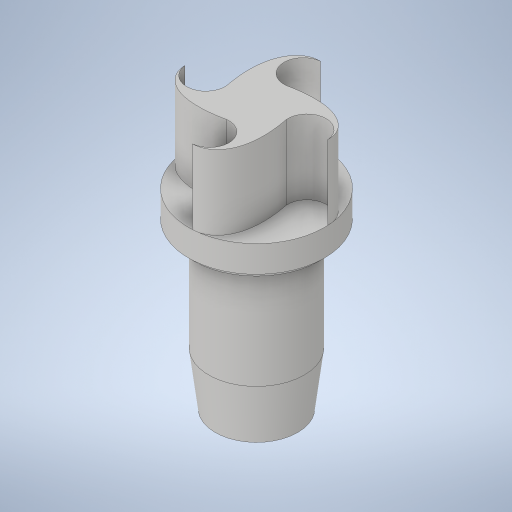
# Autodesk Inventor part: 1.3mm_uncorrected
Saved by Autodesk Inventor 2023.1 (Build 271208000, 208)
## iProperties
Created: 2020-02-22
Part Number: 1.3mm_uncorrected
Material: Générique
Document SubType Name: Modeling
Designer: kongooi
Density: 1 g/cm^3
Appearance: Par défaut
Author: kongooi
Autodesk Inventor part; units mm, degrees
ref_plane "YZ Plane" through (0, 0, 0) normal (1, 0, 0) x (0, 1, 0)
ref_plane "XZ Plane" through (0, 0, 0) normal (0, 1, 0) x (-1, 0, 0)
ref_plane "XY Plane" through (0, 0, 0) normal (0, 0, 1) x (1, 0, 0)
sketch "Sketch2" plane through (0, 0, 0) normal (0, 1, 0) x (-1, 0, 0)
  line L0 (-0.279026, 0.279026) -> (0.279026, -0.279026) construction
  line L1 (0.279026, 0.279026) -> (-0.279026, -0.279026) construction
  spline S0 degree 4 poles (-0.639115, -0.03369) (-0.634493, -0.132924) (-0.626677, -0.000796) (-0.683231, -0.424589) (0.000022, -0.278707) knots 0 0 0 0 0 1 1 1 1 1
  spline S1 degree 4 poles (0.036579, -0.638954) (0.128591, -0.633029) (0.015735, -0.629627) (0.410949, -0.676473) (0.279026, 0) knots 0 0 0 0 0 1 1 1 1 1
  spline S2 degree 4 poles (-0.036525, 0.638959) (-0.129118, 0.634798) (-0.010002, 0.617131) (-0.415936, 0.686883) (-0.279026, 0) knots 0 0 0 0 0 1 1 1 1 1
  spline S3 degree 4 poles (0.638959, 0.036525) (0.634795, 0.128622) (0.619543, 0.004623) (0.682049, 0.421677) (0, 0.279026) knots 0 0 0 0 0 1 1 1 1 1
  arc A0 (-0.639115, -0.03369) -> (-0.279026, 0) centre (-0.45907, -0.016845) ccw
  arc A1 (0.036579, -0.638954) -> (0.000022, -0.278707) centre (0.0183, -0.45883) ccw
  arc A2 (0.638959, 0.036525) -> (0.279026, 0) centre (0.458993, 0.018263) ccw
  arc A3 (-0.036525, 0.638959) -> (0, 0.279026) centre (-0.018263, 0.458993) ccw
  circle A4 centre (0, 0) radius 0.64
  point P0 (0.072027, -0.636054)
  point P1 (0.088403, -0.633939)
  point P2 (0.119628, -0.625229)
  point P3 (-0.071713, 0.635654)
  point P4 (-0.087466, 0.632637)
  point P5 (-0.11823, 0.62326)
  point P6 (0.635846, 0.070961)
  point P7 (0.633021, 0.08595)
  point P8 (0.62382, 0.11598)
  point P9 (-0.636387, -0.071601)
  point P10 (-0.634237, -0.087213)
  point P11 (-0.625654, -0.117837)
  dimension "d14" = 1.28
  constraints: 8 point on circle, 4 centre point, 4 end point, 2 midpoint, 1 coincident, 31 other
sketch "Sketch2 outline for Extrusion1" plane through (0, 0, 0) normal (0, 1, 0) x (-1, 0, 0)
  arc A0 (-0.639115, -0.03369) -> (-0.279026, 0) centre (-0.45907, -0.016845) ccw
  spline S0 degree 4 poles (-0.036525, 0.638959) (-0.129118, 0.634798) (-0.010002, 0.617131) (-0.415936, 0.686883) (-0.279026, 0) knots 0 0 0 0 0 1 1 1 1 1
  arc A1 (-0.036525, 0.638959) -> (0, 0.279026) centre (-0.018263, 0.458993) ccw
  spline S1 degree 4 poles (0.638959, 0.036525) (0.634795, 0.128622) (0.619543, 0.004623) (0.682049, 0.421677) (0, 0.279026) knots 0 0 0 0 0 1 1 1 1 1
  arc A2 (0.638959, 0.036525) -> (0.279026, 0) centre (0.458993, 0.018263) ccw
  spline S2 degree 4 poles (0.036579, -0.638954) (0.128591, -0.633029) (0.015735, -0.629627) (0.410949, -0.676473) (0.279026, 0) knots 0 0 0 0 0 1 1 1 1 1
  arc A3 (0.036579, -0.638954) -> (0.000022, -0.278707) centre (0.0183, -0.45883) ccw
  spline S3 degree 4 poles (-0.639115, -0.03369) (-0.634493, -0.132924) (-0.626677, -0.000796) (-0.683231, -0.424589) (0.000022, -0.278707) knots 0 0 0 0 0 1 1 1 1 1
extrude "Extrusion1" add sketch "Sketch2 outline for Extrusion1" along normal blind 0.7
sketch "Sketch5" plane through (0, 0, 0) normal (0, -1, 0) x (1, 0, 0)
  circle A0 centre (0.000002, 0) radius 0.64
  point P0 (0.639115, -0.03369)
  dimension "d15" = 1.28
  constraints: 3 other
extrude "Extrusion2" add sketch "Sketch5" along normal blind 0.3 separate body
sketch "Sketch6" plane through (0.000002, -0.3, 0) normal (0, -1, 0) x (1, 0, 0)
  circle A0 centre (-0.000002, 0) radius 0.45
  circle A1 centre (-0.000002, 0) radius 0.25
  dimension "d6" = 0.5
  dimension "d7" = 0.9
  constraints: 2 centre point, 2 coincident
  measures "d6" diameter of A1
  measures "d7" diameter of A0
extrude "Extrusion3" add sketch "Sketch6" along normal blind 1.5 contours A0 | A1 bodies 2
chamfer "Chanfrein1" distance 0.5 angle 7 1 edges at (-0.45, -1.8, 0) measured on face at (0.4485, -1.3, -0.0362)
chamfer "Chanfrein2" distance 0.05 angle 45 1 edges at (-0.64, -0.3, 0)
body "Solid2"
body "Solid3"
